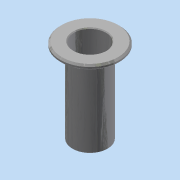
# Autodesk Inventor part: douille
Saved by Autodesk Inventor 2017 (Build 210142000, 142)
## iProperties
Created: 2018-04-15
Part Number: douille
Material: S235JR (E24-2)
Document SubType Name: Modeling
Designer: RozierB
Density: 7.85 g/cm^3
Appearance: Acier
Author: RozierB
Autodesk Inventor part; units mm, degrees
ref_plane "YZ Plane" through (0, 0, 0) normal (1, 0, 0) x (0, 1, 0)
ref_plane "XZ Plane" through (0, 0, 0) normal (0, 1, 0) x (-1, 0, 0)
ref_plane "XY Plane" through (0, 0, 0) normal (0, 0, 1) x (1, 0, 0)
sketch "Esquisse3" plane through (0, 0, 0) normal (1, 0, 0) x (0, 1, 0)
  line L0 (18.5, -1) -> (18.5, -2)
  line L1 (18.5, -2) -> (17.5, -3)
  line L2 (17.5, -3) -> (11.25, -3)
  line L3 (11.25, -3) -> (11, -3.25)
  line L4 (11, -3.25) -> (11, -52.75)
  line L5 (11, -52.75) -> (10.75, -53)
  line L6 (10.75, -53) -> (10.25, -53)
  line L7 (10.25, -53) -> (10, -52.75)
  line L8 (10, -52.75) -> (10, -0.5)
  line L9 (10, -0.5) -> (10.5, 0)
  line L10 (10.5, 0) -> (17.5, 0)
  line L11 (17.5, 0) -> (18.5, -1)
  line L12 (0, -63.6) -> (0, 10.6) projected
  point P0 (0, 0)
  dimension "d4" = 1
  dimension "d5" = 1
  dimension "d6" = 18.5
  dimension "d7" = 11
  dimension "d9" = 3
  dimension "d10" = 0.25
  dimension "d11" = 0.25
  dimension "d12" = 0.25
  dimension "d13" = 0.25
  dimension "d14" = 1
  dimension "d15" = 0.5
  dimension "d16" = 0.5
  dimension "d17" = 0.25
  dimension "d18" = 0.25
  dimension "d19" = 1
  dimension "d20" = 1
  dimension "d23" = 50
  constraints: 24 end point, 3 horizontal, 3 vertical, 1 horizontal alignment
  measures "d4" horizontal distance of L10.end L0.start
  measures "d5" horizontal distance of L10.end L0.start
  measures "d6" distance from line of point (0, 0) L0
  measures "d7" distance from line of point (0, 0) L4
  measures "d9" distance between parallel lines of L2 L10
  measures "d10" horizontal distance of L4.end L5.end
  measures "d11" horizontal distance of L4.end L5.end
  measures "d12" horizontal distance of L6.end L7.end
  measures "d13" horizontal distance of L6.end L7.end
  measures "d14" distance between parallel lines of L4 L8
  measures "d15" horizontal distance of L8.end L9.end
  measures "d16" horizontal distance of L8.end L9.end
  measures "d17" horizontal distance of L2.end L3.end
  measures "d18" horizontal distance of L2.end L3.end
  measures "d19" horizontal distance of L0.end L1.end
  measures "d20" horizontal distance of L0.end L1.end
  measures "d23" distance between parallel lines of L6 L2
revolve "Révolution1" add sketch "Esquisse3" angle 360 about axis through (0, 0, -10) along (0, 0, 1)
equation "\"d5\" = d4"
equation "\"d11\" = d10"
equation "\"d12\" = d10"
equation "\"d13\" = d10"
equation "\"d16\" = d15"
equation "\"d17\" = d10"
equation "\"d18\" = d10"
equation "\"d19\" = d4"
equation "\"d20\" = d4"
